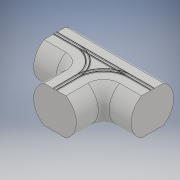
# Autodesk Inventor part: T corridor
Saved by Autodesk Inventor 2017 (Build 210142000, 142)
## iProperties
Created: 2018-03-04
Part Number: T corridor
Material: Generic
Document SubType Name: Modeling
Designer: Braxton
Density: 1 g/cm^3
Appearance: Default
Author: Braxton
Autodesk Inventor part; units mm, degrees
ref_plane "YZ Plane" through (0, 0, 0) normal (1, 0, 0) x (0, 1, 0)
ref_plane "XZ Plane" through (0, 0, 0) normal (0, 1, 0) x (-1, 0, 0)
sketch "Sketch1" plane through (0, 0, 0) normal (1, 0, 0) x (0, 1, 0)
  arc A0 (86.254167, -7.408333) -> (84.666667, -8.995833) centre (86.254167, -8.995833) ccw
  line L0 (84.666667, -8.995833) -> (84.666667, -50.8)
  arc A1 (84.666667, -4.103437) -> (86.913229, -6.35) centre (86.913229, -4.103437) ccw
  line L1 (87.843165, -6.35) -> (86.913229, -6.35)
  line L2 (87.843165, -7.408333) -> (86.254167, -7.408333)
  line L3 (84.668165, -6.348501) -> (87.843165, -3.173502) construction
  arc A2 (87.843165, -6.35) -> (84.666667, -3.173502) centre (84.668165, -6.348501) ccw construction
  line L4 (84.666667, -4.103437) -> (84.666667, 0)
  line L5 (84.666667, 0) -> (87.843165, 0) construction
  line L6 (87.843165, -6.35) -> (87.843165, 0) construction
  arc A3 (84.666667, 50.8) -> (-84.666667, 50.8) centre (0, 0) ccw
  arc A4 (-84.666667, -50.8) -> (84.666667, -50.8) centre (0, 0) ccw
  line L7 (-84.666667, 50.8) -> (-84.666667, -50.8)
  line L8 (87.843166, 7.408333) -> (86.254167, 7.408333)
  line L9 (84.666667, 8.995833) -> (84.666667, -8.995833) construction
  arc A5 (84.666667, 8.995833) -> (86.254167, 7.408333) centre (86.254167, 8.995833) ccw
  line L10 (84.666667, 4.103437) -> (84.666667, 0)
  line L11 (87.843165, 6.35) -> (87.843165, 0) construction
  line L12 (84.668165, 6.348501) -> (87.843165, 3.173502) construction
  arc A6 (84.666667, 3.173502) -> (87.843165, 6.35) centre (84.668165, 6.348501) ccw construction
  arc A7 (86.913229, 6.35) -> (84.666667, 4.103437) centre (86.913229, 4.103437) ccw
  line L13 (87.843165, 6.35) -> (86.913229, 6.35)
  line L14 (84.666667, 8.995833) -> (84.666667, 50.8)
  line L15 (87.843165, -7.408333) -> (87.843165, -6.35)
  line L16 (87.843165, 6.35) -> (87.843166, 7.408333)
  dimension "d187" = 101.6
  dimension "d188" = 14.81667
  dimension "d189" = 98.73745
  dimension "d190" = 98.73745
  dimension "d191" = 43.39167
  dimension "d192" = 1.5875
  dimension "d193" = 1.5875
  dimension "d194" = 41.80417
  dimension "d195" = 6.35
  dimension "d196" = 3.175
  dimension "d198" = 2.24656
  dimension "d199" = 45
  dimension "d200" = 84.66667
  constraints: 34 end point, 19 point on circle, 8 centre point, 7 symmetric about line, 6 point on line, 5 tangent, 4 collinear, 4 perpendicular, 3 coincident, 2 vertical, 1 equal length, 1 equal radius, 1 parallel, 3 other
  measures "d187" distance of L14.end L0.end
  measures "d188" distance of L8.start L2.start
  measures "d189" radius of A3
  measures "d190" radius of A4
  measures "d191" distance from line of L14.end L8
  measures "d192" distance from line of L0.start L2
  measures "d193" radius of A0
  measures "d194" distance of L0.start L0.end
  measures "d195" distance of L5.end L11.start
  measures "d196" distance of L11.start L12.start
  measures "d198" horizontal distance of L10.start L13.end
  measures "d199" angle of L11 L12
  measures "d200" distance from line of L7 point (0, 0)
extrude "corridor" add sketch "Sketch1" against normal blind 101.6
ref_plane "Work Plane1" through (0, 0, -124.137452) normal (0, 0, 1) x (1, 0, 0)
sketch "Sketch4" plane through (0, 0, -124.137452) normal (0, 0, 1) x (1, 0, 0)
  line L0 (0, 0) -> (124.137453, 0) construction
  line L1 (0, -84.666667) -> (0, 84.666667)
  line L2 (73.337453, -84.666667) -> (174.937453, -84.666667)
  arc A0 (73.337453, 84.666667) -> (73.337453, -84.666667) centre (124.137453, 0) ccw
  arc A1 (174.937453, -84.666667) -> (174.937453, 84.666667) centre (124.137453, 0) ccw
  line L3 (124.137453, 84.670027) -> (124.137453, 87.843165) construction
  line L4 (116.72912, 87.843165) -> (116.72912, 86.254167)
  line L5 (131.545786, 87.843165) -> (131.545786, 86.254167)
  line L6 (133.133286, 84.666667) -> (174.937453, 84.666667)
  line L7 (115.14162, 84.666667) -> (133.133286, 84.666667) construction
  arc A2 (131.545786, 86.254167) -> (133.133286, 84.666667) centre (133.133286, 86.254167) ccw
  arc A3 (115.14162, 84.666667) -> (116.72912, 86.254167) centre (115.14162, 86.254167) ccw
  line L8 (115.14162, 84.666667) -> (73.337453, 84.666667)
  line L9 (124.137453, 84.666667) -> (124.137453, 87.843165) construction
  line L10 (130.487453, 87.843165) -> (124.137453, 87.843165) construction
  line L11 (130.485954, 84.668165) -> (127.310955, 87.843165) construction
  arc A4 (130.487453, 87.843165) -> (127.310955, 84.666667) centre (130.485954, 84.668165) ccw construction
  arc A5 (128.24089, 84.666667) -> (130.487453, 86.913229) centre (128.24089, 86.913229) ccw
  line L12 (130.487453, 87.843165) -> (130.487453, 86.913229)
  line L13 (120.034016, 84.666667) -> (124.137453, 84.666667)
  line L14 (117.788952, 84.668165) -> (120.963951, 87.843165) construction
  line L15 (117.787453, 87.843165) -> (117.787453, 86.913229)
  line L16 (117.787453, 87.843165) -> (124.137453, 87.843165) construction
  arc A6 (117.787453, 86.913229) -> (120.034016, 84.666667) centre (120.034016, 86.913229) ccw
  arc A7 (120.963951, 84.666667) -> (117.787453, 87.843165) centre (117.788952, 84.668165) ccw construction
  line L17 (128.24089, 84.666667) -> (124.137453, 84.666667)
  line L18 (131.545786, 87.843165) -> (130.487453, 87.843165)
  line L19 (117.787453, 87.843165) -> (116.72912, 87.843165)
  dimension "d171" = 124.13745
  dimension "d202" = 101.6
  dimension "d203" = 14.81667
  dimension "d204" = 98.73745
  dimension "d205" = 98.73745
  dimension "d206" = 43.39167
  dimension "d207" = 1.5875
  dimension "d208" = 1.5875
  dimension "d209" = 41.80417
  dimension "d210" = 6.35
  dimension "d211" = 3.175
  dimension "d213" = 2.24656
  dimension "d214" = 45
  dimension "d215" = 84.66667
  constraints: 38 end point, 19 point on circle, 10 symmetric about line, 8 centre point, 6 point on line, 4 coincident, 4 collinear, 4 perpendicular, 3 horizontal, 3 tangent, 1 midpoint, 1 parallel, 1 vertical, 3 other
  measures "d171" distance of L0.start L0.end
  measures "d202" distance of L8.end L6.end
  measures "d203" distance of L4.start L5.start
  measures "d204" radius of A0
  measures "d205" radius of A1
  measures "d206" distance from line of L8.end L4
  measures "d207" distance from line of L6.start L5
  measures "d208" radius of A2
  measures "d209" distance of L6.start L6.end
  measures "d210" distance of L10.end L15.start
  measures "d211" distance of L15.start L14.start
  measures "d213" horizontal distance of L13.start L15.end
  measures "d214" angle of L16 L14
  measures "d215" distance from line of L2 point (124.137, 0)
extrude "T bottom" add sketch "Sketch4" against normal blind 101.6
sketch "Sketch8" plane through (0, 0, 0) normal (1, 0, 0) x (0, 0, -1)
  arc A0 (-8.995833, 84.666667) -> (-7.408333, 86.254167) centre (-8.995833, 86.254167) ccw
  line L0 (-7.408333, 87.843166) -> (-6.35, 87.843165)
  line L1 (-7.408333, 86.254167) -> (-7.408333, 87.843166)
  line L2 (-7.408333, 87.843166) -> (-6.35, 87.843165)
  arc A1 (-6.35, 86.913229) -> (-4.103437, 84.666667) centre (-4.103437, 86.913229) ccw
  line L3 (-6.35, 87.843165) -> (-6.35, 86.913229)
  arc A2 (4.103437, 84.666667) -> (6.35, 86.913229) centre (4.103437, 86.913229) ccw
  line L4 (-4.103437, 84.666667) -> (4.103437, 84.666667)
  line L5 (6.35, 87.843165) -> (7.408333, 87.843165)
  line L6 (6.35, 86.913229) -> (6.35, 87.843165)
  line L7 (6.35, 87.843165) -> (7.408333, 87.843165)
  line L8 (7.408333, 87.843165) -> (7.408333, 86.254167)
  line L9 (7.408333, 87.843165) -> (7.408333, 86.254167)
  arc A3 (7.408333, 86.254167) -> (8.995833, 84.666667) centre (8.995833, 86.254167) ccw
  arc A4 (50.8, -84.666667) -> (50.8, 84.666667) centre (0, 0) ccw
  line L10 (8.995833, 84.666667) -> (50.8, 84.666667)
  line L11 (50.8, 84.666667) -> (8.995833, 84.666667)
  line L12 (-8.995833, 84.666667) -> (-8.995833, -84.666667)
  line L13 (50.8, -84.666667) -> (-50.8, -84.666667)
  line L14 (-8.995833, -84.666667) -> (50.8, -84.666667)
  arc A5 (50.8, -84.666667) -> (50.8, 84.666667) centre (0, 0) ccw
  arc A6 (7.408333, 86.254167) -> (8.995833, 84.666667) centre (8.995833, 86.254167) ccw
  arc A7 (4.103437, 84.666667) -> (6.35, 86.913229) centre (4.103437, 86.913229) ccw
  arc A8 (-6.35, 86.913229) -> (-4.103437, 84.666667) centre (-4.103437, 86.913229) ccw
  arc A9 (-8.995833, 84.666667) -> (-7.408333, 86.254167) centre (-8.995833, 86.254167) ccw
  arc A10 (7.408333, 86.254167) -> (8.995833, 84.666667) centre (8.995833, 86.254167) ccw
  constraints: 20 end point, 10 point on circle, 5 centre point, 5 perpendicular, 4 collinear, 3 concentric, 3 tangent, 1 point on line, 1 vertical
sketch "Sketch7" plane through (0, 0, 0) normal (0, 1, 0) x (-1, 0, 0)
  arc A0 (0, -98.737452) -> (-25.400001, -124.137452) centre (0, -124.137453) ccw
  line L0 (-25.400001, -124.137452) -> (-25.400004, -212.884054) construction
  line L1 (0, -98.737452) -> (101.6, -98.737452) construction
  line L2 (-25.400001, -124.137452) -> (-25.400001, -225.737452)
  line L3 (-222.874905, -124.137452) -> (-222.874905, -225.737452) construction
  arc A1 (-222.874905, -124.137452) -> (-248.274905, -98.737452) centre (-248.274905, -124.137452) ccw
  line L4 (-248.274905, -98.737452) -> (-387.354408, -98.737452) construction
  point P0 (0, 0)
  constraints: 6 end point, 5 point on circle, 4 tangent, 2 centre point, 1 collinear, 1 point on line
sweep "corner curve" add profiles "Sketch8" path "Sketch7" path curves A0
sketch "Sketch9" plane through (0, 0, 0) normal (1, 0, 0) x (0, 0, -1)
  arc A0 (-8.995833, 84.666667) -> (-7.408333, 86.254167) centre (-8.995833, 86.254167) ccw
  arc A1 (-50.8, 84.666667) -> (-50.8, -84.666667) centre (0, 0) ccw
  line L0 (-50.8, 84.666667) -> (-8.995833, 84.666667)
  line L1 (-50.8, 84.666667) -> (-8.995833, 84.666667)
  arc A2 (-50.8, 84.666667) -> (-50.8, -84.666667) centre (0, 0) ccw
  arc A3 (7.408333, 86.254167) -> (8.995833, 84.666667) centre (8.995833, 86.254167) ccw
  line L2 (7.408333, 87.843165) -> (7.408333, 86.254167)
  line L3 (7.408333, 86.254167) -> (7.408333, 87.843165)
  line L4 (6.35, 87.843165) -> (7.408333, 87.843165)
  line L5 (7.408333, 87.843165) -> (6.35, 87.843165)
  line L6 (6.35, 86.913229) -> (6.35, 87.843165)
  line L7 (6.35, 87.843165) -> (6.35, 86.913229)
  line L8 (-4.103437, 84.666667) -> (4.103437, 84.666667)
  line L9 (4.103437, 84.666667) -> (-4.103437, 84.666667)
  arc A4 (-6.35, 86.913229) -> (-4.103437, 84.666667) centre (-4.103437, 86.913229) ccw
  line L10 (-7.408333, 87.843166) -> (-6.35, 87.843165)
  line L11 (-6.35, 86.913229) -> (-6.35, 87.843165)
  line L12 (-6.35, 87.843165) -> (-7.408333, 87.843166)
  line L13 (-7.408333, 87.843166) -> (-7.408333, 86.254167)
  arc A5 (7.408333, 86.254167) -> (8.995833, 84.666667) centre (8.995833, 86.254167) ccw
  arc A6 (4.103437, 84.666667) -> (6.35, 86.913229) centre (4.103437, 86.913229) ccw
  arc A7 (4.103437, 84.666667) -> (6.35, 86.913229) centre (4.103437, 86.913229) ccw
  line L14 (-6.35, 87.843165) -> (-6.35, 86.913229)
  arc A8 (-6.35, 86.913229) -> (-4.103437, 84.666667) centre (-4.103437, 86.913229) ccw
  arc A9 (-8.995833, 84.666667) -> (-7.408333, 86.254167) centre (-8.995833, 86.254167) ccw
  line L15 (8.995833, 84.666667) -> (8.995833, -84.666667)
  line L16 (50.8, -84.666667) -> (-50.8, -84.666667)
  line L17 (-50.8, -84.666667) -> (8.995833, -84.666667)
  constraints: 20 end point, 10 point on circle, 5 centre point, 5 concentric, 5 perpendicular, 3 collinear, 1 horizontal, 1 point on line, 1 vertical
extrude "flat of T" add sketch "Sketch9" along normal blind 124.137452
mirror "Mirror parts" about plane through (124.137452, 1.268005, 30.174282) normal (1, 0, 0) of "flat of T", "corridor"
sketch "Sketch17" plane through (0, 0, -124.137452) normal (0, 0, 1) x (1, 0, 0)
  line L0 (116.72912, 86.254167) -> (116.72912, 87.843165)
  line L1 (116.72912, 86.254167) -> (116.72912, 87.843165)
  line L2 (116.72912, 87.843165) -> (117.787453, 87.843165)
  line L3 (116.72912, 87.843165) -> (117.787453, 87.843165)
  line L4 (117.787453, 87.843165) -> (117.787453, 86.913229)
  line L5 (117.787453, 87.843165) -> (117.787453, 86.913229)
  line L6 (120.034016, 84.666667) -> (128.24089, 84.666667)
  arc A0 (128.24089, 84.666667) -> (130.487453, 86.913229) centre (128.24089, 86.913229) ccw
  line L7 (120.034016, 84.666667) -> (128.24089, 84.666667)
  line L8 (130.487453, 86.913229) -> (130.487453, 87.843165)
  line L9 (130.487453, 86.913229) -> (130.487453, 87.843165)
  line L10 (130.487453, 87.843165) -> (131.545786, 87.843165)
  line L11 (130.487453, 87.843165) -> (131.545786, 87.843165)
  line L12 (131.545786, 87.843165) -> (131.545786, 86.254167)
  line L13 (131.545786, 87.843165) -> (131.545786, 86.254167)
  arc A1 (131.545786, 86.254167) -> (133.133286, 84.666667) centre (133.133286, 86.254167) ccw
  arc A2 (174.937453, -84.666667) -> (174.937453, 84.666667) centre (124.137453, 0) ccw
  line L14 (133.133286, 84.666667) -> (174.937453, 84.666667)
  line L15 (174.937453, 84.666667) -> (133.133286, 84.666667)
  arc A3 (115.14162, 84.666667) -> (116.72912, 86.254167) centre (115.14162, 86.254167) ccw
  line L16 (115.14162, 84.666667) -> (115.14162, -84.666667)
  line L17 (174.937453, -84.666667) -> (73.337453, -84.666667)
  line L18 (115.14162, -84.666667) -> (174.937453, -84.666667)
  arc A4 (174.937453, -84.666667) -> (174.937453, 84.666667) centre (124.137453, 0) ccw
  arc A5 (115.14162, 84.666667) -> (116.72912, 86.254167) centre (115.14162, 86.254167) ccw
  arc A6 (117.787453, 86.913229) -> (120.034016, 84.666667) centre (120.034016, 86.913229) ccw
  arc A7 (128.24089, 84.666667) -> (130.487453, 86.913229) centre (128.24089, 86.913229) ccw
  arc A8 (131.545786, 86.254167) -> (133.133286, 84.666667) centre (133.133286, 86.254167) ccw
  arc A9 (117.787453, 86.913229) -> (120.034016, 84.666667) centre (120.034016, 86.913229) ccw
  point P0 (0, 0)
  constraints: 20 end point, 11 point on circle, 5 centre point, 5 collinear, 4 concentric, 2 perpendicular, 2 tangent, 2 vertical, 1 coincident, 1 horizontal, 1 point on line
sweep "corner curve 2" add profiles "Sketch17" path "Sketch7" path curves A1
sketch "Sketch19" plane through (133.133286, 84.666667, -225.737452) normal (0, 1, 0) x (1, 0, 0)
  line L0 (-66.29857, -216.741619) -> (48.306902, -216.741619)
  arc A0 (-66.29857, -216.741619) -> (-8.995833, -149.707844) centre (-133.133286, -101.599999) ccw
  line L1 (48.306902, -216.741619) -> (-66.29857, -216.741619)
  arc A1 (-8.995833, -149.707844) -> (48.306902, -216.741619) centre (115.141619, -101.6) ccw
  arc A2 (-66.29857, -216.741619) -> (-8.995833, -149.707844) centre (-133.133286, -101.599999) ccw
  arc A3 (-8.995833, -149.707844) -> (48.306902, -216.741619) centre (115.141619, -101.6) ccw
  arc A4 (-8.995833, -149.707844) -> (48.306902, -216.741619) centre (115.141619, -101.6) ccw
  point P0 (-133.133286, -225.737452)
  constraints: 4 point on circle, 2 centre point, 2 concentric, 2 end point, 1 horizontal
extrude "hole fill in" add sketch "Sketch19" against normal up to surface (169.333333 mm away)
equation "\"d5\" = -0.5 * d2"
equation "\"d2\" = 248.274904"
body "Solid1"
